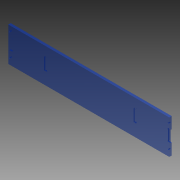
# Autodesk Inventor part: shelfTop
Saved by Autodesk Inventor 2015 SP1 (Build 190203100, 203)
## iProperties
Created: 2015-04-10
Part Number: shelfTop
Material: Generic
Document SubType Name: Modeling
Designer: Iain
Density: 1 g/cm^3
Appearance: Clear - Blue
Author: Iain
Autodesk Inventor part; units mm, degrees
ref_plane "YZ Plane" through (0, 0, 0) normal (1, 0, 0) x (0, 1, 0)
sketch "Sketch1" plane through (0, 0, 0) normal (0, 1, 0) x (-1, 0, 0)
  line L0 (590, -125) -> (-590, -125)
  line L1 (-590, -125) -> (-590, 125)
  line L2 (-590, 125) -> (590, 125)
  line L3 (590, 125) -> (590, -125)
  point P0 (0, 0)
  point P1 (0, 125)
  point P2 (-590, 0)
  dimension "d0" = 250
  dimension "d1" = 1180
  constraints: 8 end point, 2 midpoint, 2 parallel, 1 horizontal, 1 horizontal alignment, 1 perpendicular, 1 vertical alignment
  measures "d0" distance of L2.end L0.start
  measures "d1" distance of L0.start L0.end
extrude "Extrusion1" add sketch "Sketch1" along normal blind 18
sketch "Sketch2" plane through (0, 18, 0) normal (0, 1, 0) x (1, 0, 0)
  line L0 (590, 125) -> (-590, 125) projected
  line L1 (-590, 125) -> (-590, -125) projected
  line L2 (-590, -125) -> (590, -125) projected
  line L3 (590, -125) -> (590, 125) projected
  line L4 (-590, 41.6667) -> (-572, 41.6667)
  line L5 (-572, 41.6667) -> (-572, -41.6667)
  line L6 (-572, -41.6667) -> (-590, -41.6667)
  line L7 (-590, -41.6667) -> (-590, 41.6667)
  line L8 (-590, 125) -> (-590, -125) projected
  point P0 (0, 0)
  point P1 (-572, 0)
  point P2 (-590, 0)
  point P3 (-590, 0)
  point P4 (-590, 0)
  dimension "d4" = 18
  dimension "d5" = 83.3333
  constraints: 8 end point, 4 midpoint, 2 parallel, 1 coincident, 1 horizontal, 1 horizontal alignment, 1 perpendicular
  measures "d4" distance of L4.start L4.end
  measures "d5" distance of L6.end L4.start
extrude "Extrusion2" cut sketch "Sketch2" against normal blind 9 contours L4 L5 L6 L1
ref_plane "Work Plane1" through (0, 0, 125) normal (-1, 0, 0) x (0, 0, 1)
mirror "Mirror1" about plane through (0, 0, 125) normal (-1, 0, 0) of "Extrusion2"
sketch "Sketch3" plane through (0, 18, 0) normal (0, 1, 0) x (1, 0, 0)
  line L0 (590, -41.6667) -> (572, -41.6667) projected
  line L1 (572, -41.6667) -> (572, 41.6667) projected
  line L2 (572, 41.6667) -> (590, 41.6667) projected
  line L3 (590, 41.6667) -> (590, 125) projected
  line L4 (590, 125) -> (-590, 125) projected
  line L5 (-590, 125) -> (-590, 41.6667) projected
  line L6 (-590, 41.6667) -> (-572, 41.6667) projected
  line L7 (-572, 41.6667) -> (-572, -41.6667) projected
  line L8 (-572, -41.6667) -> (-590, -41.6667) projected
  line L9 (-590, -41.6667) -> (-590, -125) projected
  line L10 (-590, -125) -> (590, -125) projected
  line L11 (590, -125) -> (590, -41.6667) projected
  line L12 (-336.7778, 41.6667) -> (-318.7778, 41.6667)
  line L13 (-318.7778, 41.6667) -> (-318.7778, -41.6667)
  line L14 (-318.7778, -41.6667) -> (-336.7778, -41.6667)
  line L15 (-336.7778, -41.6667) -> (-336.7778, 41.6667)
  line L16 (-318.7778, 41.6667) -> (-327.7778, 41.6667) construction
  point P0 (0, 0)
  point P1 (-318.7778, 0)
  point P2 (-572, 0)
  point P3 (-323.2778, 41.6667)
  point P4 (-327.7778, 41.6667)
  dimension "d9" = 18
  dimension "d10" = 83.3333
  dimension "d11" = 83.3333
  dimension "d15" = 9
  dimension "d16" = 262.2222
  constraints: 10 end point, 4 midpoint, 2 horizontal, 2 horizontal alignment, 2 parallel, 1 coincident, 1 perpendicular
  measures "d9" distance of L12.start L12.end
  measures "d10" distance of L12.end L13.end
  measures "d11" distance of L6.end L7.end
  measures "d15" distance of L16.start L16.end
  measures "d16" horizontal distance of L4.end L16.end
extrude "Extrusion3" cut sketch "Sketch3" against normal blind 9 contours L12 L13 L14 L15
mirror "Mirror2" about plane through (0, 0, 125) normal (-1, 0, 0) of "Extrusion3"
sketch "Sketch4" plane through (0, 18, 0) normal (0, 1, 0) x (1, 0, 0)
  line L0 (336.7778, 41.6667) -> (336.7778, -41.6667) projected
  line L1 (336.7778, -41.6667) -> (318.7778, -41.6667) projected
  line L2 (318.7778, -41.6667) -> (318.7778, 41.6667) projected
  line L3 (318.7778, 41.6667) -> (336.7778, 41.6667) projected
  line L4 (-336.7778, -41.6667) -> (-336.7778, 41.6667) projected
  line L5 (-336.7778, 41.6667) -> (-318.7778, 41.6667) projected
  line L6 (-318.7778, 41.6667) -> (-318.7778, -41.6667) projected
  line L7 (-318.7778, -41.6667) -> (-336.7778, -41.6667) projected
  line L8 (590, -41.6667) -> (572, -41.6667) projected
  line L9 (572, -41.6667) -> (572, 41.6667) projected
  line L10 (572, 41.6667) -> (590, 41.6667) projected
  line L11 (590, 41.6667) -> (590, 125) projected
  line L12 (590, 125) -> (-590, 125) projected
  line L13 (-590, 125) -> (-590, 41.6667) projected
  line L14 (-590, 41.6667) -> (-572, 41.6667) projected
  line L15 (-572, 41.6667) -> (-572, -41.6667) projected
  line L16 (-572, -41.6667) -> (-590, -41.6667) projected
  line L17 (-590, -41.6667) -> (-590, -125) projected
  line L18 (-590, -125) -> (590, -125) projected
  line L19 (590, -125) -> (590, -41.6667) projected
  point P0 (0, 0)
  point P1 (572, -38.4917)
  dimension "d17" = 3.175
  constraints: 1 vertical alignment
  measures "d17" distance from line of L8 point (572, -38.492)
hole "Hole1" at (572, 18, 38.4917) direction (0, -1, 0) diameter 6.35 depth 9 tip angle 118
ref_plane "Work Plane2" through (590, 9, 0) normal (0, 0, -1) x (-1, 0, 0)
mirror "Mirror3" about plane through (590, 9, 0) normal (0, 0, -1) of "Hole1"
mirror "Mirror4" about plane through (0, 0, 125) normal (-1, 0, 0) of "Hole1", "Mirror3"
sketch "Sketch5" plane through (318.7778, 9, -41.6667) normal (0, 1, 0) x (1, 0, 0)
  line L0 (18, 0) -> (18, -83.3333) projected
  line L1 (18, -83.3333) -> (0, -83.3333) projected
  line L2 (0, -83.3333) -> (0, 0) projected
  line L3 (0, 0) -> (18, 0) projected
  line L4 (-655.5556, -83.3333) -> (-655.5556, 0) projected
  line L5 (-655.5556, 0) -> (-637.5556, 0) projected
  line L6 (-637.5556, 0) -> (-637.5556, -83.3333) projected
  line L7 (-637.5556, -83.3333) -> (-655.5556, -83.3333) projected
  arc A0 (-890.7778, -6.35) -> (-890.7778, 0) centre (-890.7778, -3.175) ccw projected
  line L8 (-890.7778, -6.35) -> (-890.7778, -76.9833) projected
  arc A1 (-890.7778, -83.3333) -> (-890.7778, -76.9833) centre (-890.7778, -80.1583) ccw projected
  line L9 (-890.7778, -83.3333) -> (-908.7778, -83.3333) projected
  line L10 (-908.7778, -83.3333) -> (-908.7778, -166.6667) projected
  line L11 (-908.7778, -166.6667) -> (271.2222, -166.6667) projected
  line L12 (271.2222, -166.6667) -> (271.2222, -83.3333) projected
  line L13 (271.2222, -83.3333) -> (253.2222, -83.3333) projected
  arc A2 (253.2222, -76.9833) -> (253.2222, -83.3333) centre (253.2222, -80.1583) ccw projected
  line L14 (253.2222, -76.9833) -> (253.2222, -6.35) projected
  arc A3 (253.2222, 0) -> (253.2222, -6.35) centre (253.2222, -3.175) ccw projected
  line L15 (253.2222, 0) -> (271.2222, 0) projected
  line L16 (271.2222, 0) -> (271.2222, 83.3333) projected
  line L17 (271.2222, 83.3333) -> (-908.7778, 83.3333) projected
  line L18 (-908.7778, 83.3333) -> (-908.7778, 0) projected
  line L19 (-908.7778, 0) -> (-890.7778, 0) projected
  point P0 (-318.7778, -41.6667)
  point P1 (14.825, -83.3333)
  point P2 (3.175, -83.3333)
  dimension "d25" = 3.175
  dimension "d26" = 3.175
  constraints: 2 horizontal alignment
  measures "d25" distance from line of L0 point (14.825, -83.333)
  measures "d26" distance from line of L2 point (3.175, -83.333)
hole "Hole2" at (333.6028, 9, 41.6667) at (321.9528, 9, 41.6667) direction (0, 1, 0) diameter 6.35 depth 9 tip angle 118
mirror "Mirror5" about plane through (590, 9, 0) normal (0, 0, -1) of "Hole2"
mirror "Mirror6" about plane through (0, 0, 125) normal (-1, 0, 0) of "Hole2", "Mirror5"
sketch "Sketch7" plane through (0, 18, 0) normal (0, 1, 0) x (1, 0, 0)
  arc A0 (336.7778, 41.6667) -> (330.4278, 41.6667) centre (333.6028, 41.6667) ccw projected
  line L0 (336.7778, 41.6667) -> (336.7778, -41.6667) projected
  arc A1 (330.4278, -41.6667) -> (336.7778, -41.6667) centre (333.6028, -41.6667) ccw projected
  line L1 (330.4278, -41.6667) -> (325.1278, -41.6667) projected
  arc A2 (318.7778, -41.6667) -> (325.1278, -41.6667) centre (321.9528, -41.6667) ccw projected
  line L2 (318.7778, -41.6667) -> (318.7778, 41.6667) projected
  arc A3 (325.1278, 41.6667) -> (318.7778, 41.6667) centre (321.9528, 41.6667) ccw projected
  line L3 (325.1278, 41.6667) -> (330.4278, 41.6667) projected
  arc A4 (-572, 35.3167) -> (-572, 41.6667) centre (-572, 38.4917) ccw projected
  line L4 (-572, 35.3167) -> (-572, -35.3167) projected
  arc A5 (-572, -41.6667) -> (-572, -35.3167) centre (-572, -38.4917) ccw projected
  line L5 (-572, -41.6667) -> (-590, -41.6667) projected
  line L6 (-590, -41.6667) -> (-590, -125) projected
  line L7 (-590, -125) -> (590, -125) projected
  line L8 (590, -125) -> (590, -41.6667) projected
  line L9 (590, -41.6667) -> (572, -41.6667) projected
  arc A6 (572, -35.3167) -> (572, -41.6667) centre (572, -38.4917) ccw projected
  line L10 (572, -35.3167) -> (572, 35.3167) projected
  arc A7 (572, 41.6667) -> (572, 35.3167) centre (572, 38.4917) ccw projected
  line L11 (572, 41.6667) -> (590, 41.6667) projected
  line L12 (590, 41.6667) -> (590, 125) projected
  line L13 (590, 125) -> (-590, 125) projected
  line L14 (-590, 125) -> (-590, 41.6667) projected
  line L15 (-590, 41.6667) -> (-572, 41.6667) projected
  arc A8 (-330.4278, 41.6667) -> (-336.7778, 41.6667) centre (-333.6028, 41.6667) ccw projected
  line L16 (-330.4278, 41.6667) -> (-325.1278, 41.6667) projected
  arc A9 (-318.7778, 41.6667) -> (-325.1278, 41.6667) centre (-321.9528, 41.6667) ccw projected
  line L17 (-318.7778, 41.6667) -> (-318.7778, -41.6667) projected
  arc A10 (-325.1278, -41.6667) -> (-318.7778, -41.6667) centre (-321.9528, -41.6667) ccw projected
  line L18 (-325.1278, -41.6667) -> (-330.4278, -41.6667) projected
  arc A11 (-336.7778, -41.6667) -> (-330.4278, -41.6667) centre (-333.6028, -41.6667) ccw projected
  line L19 (-336.7778, -41.6667) -> (-336.7778, 41.6667) projected
  point P0 (0, 0)
  point P1 (581, -83.3333)
  point P2 (581, 83.3333)
  point P3 (590, 83.3333)
  point P4 (590, -83.3333)
  dimension "d34" = 9
  dimension "d35" = 9
  constraints: 2 horizontal alignment, 2 midpoint
  measures "d34" distance of point (590, -83.333) point (581, -83.333)
  measures "d35" distance of point (590, 83.333) point (581, 83.333)
hole "Hole3" at (581, 18, 83.3333) at (581, 18, -83.3333) direction (0, -1, 0) diameter 6.35 end through all
mirror "Mirror7" about plane through (0, 0, 125) normal (-1, 0, 0) of "Hole3"
equation "\"d0\" = shelfWidth"
equation "\"d1\" = shelfLength"
equation "\"d2\" = plyThickness"
equation "\"d4\" = plyThickness"
equation "\"d5\" = 0.333333 * shelfWidth"
equation "\"d7\" = 0.5 * plyThickness"
equation "\"d9\" = plyThickness"
equation "\"d10\" = 0.333333 * shelfWidth"
equation "\"d15\" = 0.5 * plyThickness"
equation "\"d16\" = 0.222222 * shelfLength"
equation "\"d13\" = 0.5 * plyThickness"
equation "\"d17\" = 0.5 * millDiameter"
equation "\"d18\" = millDiameter"
equation "\"d23\" = 0.5 * plyThickness"
equation "\"d25\" = 0.5 * millDiameter"
equation "\"d26\" = 0.5 * millDiameter"
equation "\"d27\" = millDiameter"
equation "\"d32\" = 0.5 * plyThickness"
equation "\"d34\" = 0.5 * plyThickness"
equation "\"d35\" = 0.5 * plyThickness"
equation "\"d36\" = millDiameter"
equation "\"d41\" = 0.5 * plyThickness"
equation "\"plyThickness\" = 18"
equation "\"legHeight\" = 702"
equation "\"millDiameter\" = 6.35"
equation "\"legTopTabHeight\" = 18"
equation "\"legTopSlotDepth\" = 49"
equation "\"shelfLength\" = 1180"
equation "\"shelfWidth\" = 250"
body "Solid1"
